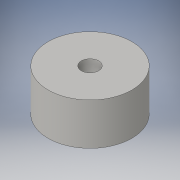
# Autodesk Inventor part: Spacer_2_00_in
Saved by Autodesk Inventor 2016 (Build 200138000, 138)
## iProperties
Created: 2015-10-18
Part Number: Spacer_2_00_in
Material: Generic
Document SubType Name: Modeling
Designer: steele
Density: 1 g/cm^3
Appearance: Default
Author: steele
Autodesk Inventor part; units mm, degrees
ref_plane "YZ Plane" through (0, 0, 0) normal (1, 0, 0) x (0, 1, 0)
ref_plane "XZ Plane" through (0, 0, 0) normal (0, 1, 0) x (-1, 0, 0)
ref_plane "XY Plane" through (0, 0, 0) normal (0, 0, 1) x (1, 0, 0)
sketch "Sketch1" plane through (0, 0, 0) normal (0, 1, 0) x (-1, 0, 0)
  circle A0 centre (0, 0) radius 10.5
  circle A1 centre (0, 0) radius 50.8
  dimension "d0" = 21
  dimension "d1" = 101.6
  constraints: 2 centre point, 2 coincident
  measures "d0" diameter of A0
  measures "d1" diameter of A1
extrude "Extrusion1" add sketch "Sketch1" along normal blind 50.8
body "Solid1"
